Autodesk Inventor part; units mm, degrees
(part 2 of 2)
sketch "Sketch26" plane through (0, 0, 0) normal (0, -1, 0) x (1, 0, 0)
  circle A0 centre (0, 0) radius 28.575 construction
  spline S0 degree 2 poles (-30.0314, 4.4782) (-29.616, 4.4453) (-29.0046, 4.0789) (-28.8177, 3.8006) knots 0 0 0 1 2 2 2
  spline S1 degree 2 poles (-28.8177, 3.8006) (-28.5989, 3.4653) (-28.4482, 2.7311) (-28.4932, 2.1623) knots 0 0 0 1 2 2 2
  line L0 (-28.4932, 2.1623) -> (-28.6199, 0.5643)
  line L1 (-28.6199, 0.5643) -> (-34.1904, 1.0057)
  line L2 (-34.1904, 1.0057) -> (-34.0734, 2.4818)
  spline S2 degree 2 poles (-34.0734, 2.4818) (-34.0262, 3.0777) (-33.9023, 3.6675) (-33.7318, 3.9265) knots 0 0 0 1 2 2 2
  spline S3 degree 2 poles (-33.7318, 3.9265) (-33.5499, 4.2165) (-33.0089, 4.4507) (-32.6568, 4.4228) knots 0 0 0 1 2 2 2
  spline S4 degree 2 poles (-32.6568, 4.4228) (-32.2641, 4.3917) (-31.674, 3.927) (-31.5269, 3.5474) knots 0 0 0 1 2 2 2
  line L3 (-31.5269, 3.5474) -> (-31.4998, 3.5453)
  spline S5 degree 2 poles (-31.4998, 3.5453) (-31.3251, 4.0311) (-30.564, 4.5204) (-30.0314, 4.4782) knots 0 0 0 1 2 2 2
  spline S6 degree 2 poles (-30.0609, 3.7038) (-30.3769, 3.7288) (-30.7975, 3.5805) (-30.9634, 3.3211) knots 0 0 0 1 2 2 2
  spline S7 degree 2 poles (-30.9634, 3.3211) (-31.0676, 3.1522) (-31.1547, 2.7411) (-31.1851, 2.3574) knots 0 0 0 1 2 2 2
  line L4 (-31.1851, 2.3574) -> (-31.2517, 1.5178)
  line L5 (-31.2517, 1.5178) -> (-29.1932, 1.3547)
  line L6 (-29.1932, 1.3547) -> (-29.1456, 1.9551)
  spline S8 degree 2 poles (-29.1456, 1.9551) (-29.107, 2.4426) (-29.1529, 3.0095) (-29.2802, 3.2377) knots 0 0 0 1 2 2 2
  spline S9 degree 2 poles (-29.2802, 3.2377) (-29.4127, 3.4571) (-29.7675, 3.6806) (-30.0609, 3.7038) knots 0 0 0 1 2 2 2
  spline S10 degree 2 poles (-32.6141, 3.6426) (-32.8128, 3.6584) (-33.1214, 3.5466) (-33.219, 3.4044) knots 0 0 0 1 2 2 2
  spline S11 degree 2 poles (-33.219, 3.4044) (-33.3326, 3.2317) (-33.4125, 2.7974) (-33.4436, 2.4047) knots 0 0 0 1 2 2 2
  line L7 (-33.4436, 2.4047) -> (-33.4997, 1.6959)
  line L8 (-33.4997, 1.6959) -> (-31.8701, 1.5668)
  line L9 (-31.8701, 1.5668) -> (-31.8036, 2.4064)
  spline S12 degree 2 poles (-31.8036, 2.4064) (-31.776, 2.754) (-31.8222, 3.0893) (-31.9211, 3.2743) knots 0 0 0 1 2 2 2
  spline S13 degree 2 poles (-31.9211, 3.2743) (-32.0158, 3.4544) (-32.3523, 3.6219) (-32.6141, 3.6426) knots 0 0 0 1 2 2 2
  spline S14 degree 2 poles (-29.4283, 8.8448) (-28.3968, 8.6022) (-27.506, 7.346) (-27.7009, 6.5173) knots 0 0 0 1 2 2 2
  spline S15 degree 2 poles (-27.7009, 6.5173) (-27.901, 5.6665) (-29.2895, 4.965) (-30.2857, 5.1993) knots 0 0 0 1 2 2 2
  spline S16 degree 2 poles (-30.2857, 5.1993) (-31.3084, 5.4398) (-32.2049, 6.7113) (-32.012, 7.5312) knots 0 0 0 1 2 2 2
  spline S17 degree 2 poles (-32.012, 7.5312) (-31.8171, 8.3599) (-30.4554, 9.0863) (-29.4283, 8.8448) knots 0 0 0 1 2 2 2
  spline S18 degree 2 poles (-29.5952, 8.1351) (-30.3887, 8.3217) (-31.2959, 7.9256) (-31.4214, 7.3923) knots 0 0 0 1 2 2 2
  spline S19 degree 2 poles (-31.4214, 7.3923) (-31.5468, 6.8589) (-30.9122, 6.0956) (-30.1188, 5.909) knots 0 0 0 1 2 2 2
  spline S20 degree 2 poles (-30.1188, 5.909) (-29.3474, 5.7275) (-28.4171, 6.1228) (-28.2916, 6.6562) knots 0 0 0 1 2 2 2
  spline S21 degree 2 poles (-28.2916, 6.6562) (-28.1672, 7.1851) (-28.8106, 7.9505) (-29.5952, 8.1351) knots 0 0 0 1 2 2 2
  spline S22 degree 2 poles (-26.6089, 10.2025) (-26.8054, 9.662) (-27.6438, 9.2779) (-28.312, 9.5208) knots 0 0 0 1 2 2 2
  line L10 (-28.312, 9.5208) -> (-30.4951, 10.3148)
  line L11 (-30.4951, 10.3148) -> (-30.6576, 9.868)
  line L12 (-30.6576, 9.868) -> (-31.2066, 10.0676)
  line L13 (-31.2066, 10.0676) -> (-31.0441, 10.5145)
  line L14 (-31.0441, 10.5145) -> (-32.1761, 10.9262)
  line L15 (-32.1761, 10.9262) -> (-31.9347, 11.5901)
  line L16 (-31.9347, 11.5901) -> (-30.8027, 11.1784)
  line L17 (-30.8027, 11.1784) -> (-30.3585, 12.3997)
  line L18 (-30.3585, 12.3997) -> (-29.8095, 12.2001)
  line L19 (-29.8095, 12.2001) -> (-30.2537, 10.9787)
  line L20 (-30.2537, 10.9787) -> (-28.3769, 10.2962)
  spline S23 degree 2 poles (-28.3769, 10.2962) (-28.079, 10.1878) (-27.7436, 10.0899) (-27.5769, 10.1112) knots 0 0 0 1 2 2 2
  spline S24 degree 2 poles (-27.5769, 10.1112) (-27.4318, 10.1259) (-27.2109, 10.3491) (-27.1273, 10.5789) knots 0 0 0 1 2 2 2
  spline S25 degree 2 poles (-27.1273, 10.5789) (-27.0685, 10.7406) (-27.0565, 11.0784) (-27.0615, 11.1573) knots 0 0 0 1 2 2 2
  line L21 (-27.0615, 11.1573) -> (-27.0476, 11.1956)
  line L22 (-27.0476, 11.1956) -> (-26.4518, 10.9789)
  spline S26 degree 2 poles (-26.4518, 10.9789) (-26.4688, 10.7731) (-26.5485, 10.3684) (-26.6089, 10.2025) knots 0 0 0 1 2 2 2
  spline S27 degree 2 poles (-25.5848, 12.5515) (-25.8291, 12.0309) (-26.6986, 11.7236) (-27.3422, 12.0256) knots 0 0 0 1 2 2 2
  line L23 (-27.3422, 12.0256) -> (-29.4452, 13.0125)
  line L24 (-29.4452, 13.0125) -> (-29.6472, 12.5821)
  line L25 (-29.6472, 12.5821) -> (-30.1761, 12.8302)
  line L26 (-30.1761, 12.8302) -> (-29.9741, 13.2607)
  line L27 (-29.9741, 13.2607) -> (-31.0645, 13.7724)
  line L28 (-31.0645, 13.7724) -> (-30.7644, 14.4119)
  line L29 (-30.7644, 14.4119) -> (-29.674, 13.9002)
  line L30 (-29.674, 13.9002) -> (-29.1219, 15.0767)
  line L31 (-29.1219, 15.0767) -> (-28.593, 14.8286)
  line L32 (-28.593, 14.8286) -> (-29.1451, 13.652)
  line L33 (-29.1451, 13.652) -> (-27.3373, 12.8037)
  spline S28 degree 2 poles (-27.3373, 12.8037) (-27.0503, 12.669) (-26.7251, 12.5414) (-26.5571, 12.5476) knots 0 0 0 1 2 2 2
  spline S29 degree 2 poles (-26.5571, 12.5476) (-26.4113, 12.5492) (-26.1712, 12.7516) (-26.0673, 12.973) knots 0 0 0 1 2 2 2
  spline S30 degree 2 poles (-26.0673, 12.973) (-25.9942, 13.1288) (-25.9519, 13.4641) (-25.9498, 13.5432) knots 0 0 0 1 2 2 2
  line L34 (-25.9498, 13.5432) -> (-25.9325, 13.58)
  line L35 (-25.9325, 13.58) -> (-25.3586, 13.3107)
  spline S31 degree 2 poles (-25.3586, 13.3107) (-25.394, 13.1073) (-25.5098, 12.7114) (-25.5848, 12.5515) knots 0 0 0 1 2 2 2
  spline S32 degree 2 poles (-25.0529, 17.7935) (-24.1532, 17.2337) (-23.711, 15.7585) (-24.1608, 15.0357) knots 0 0 0 1 2 2 2
  spline S33 degree 2 poles (-24.1608, 15.0357) (-24.6225, 14.2936) (-26.1624, 14.0731) (-27.0313, 14.6138) knots 0 0 0 1 2 2 2
  spline S34 degree 2 poles (-27.0313, 14.6138) (-27.9233, 15.1688) (-28.366, 16.6602) (-27.9211, 17.3754) knots 0 0 0 1 2 2 2
  spline S35 degree 2 poles (-27.9211, 17.3754) (-27.4713, 18.0982) (-25.9488, 18.3509) (-25.0529, 17.7935) knots 0 0 0 1 2 2 2
  spline S36 degree 2 poles (-25.4381, 17.1744) (-26.1301, 17.6051) (-27.1164, 17.52) (-27.4058, 17.0548) knots 0 0 0 1 2 2 2
  spline S37 degree 2 poles (-27.4058, 17.0548) (-27.6953, 16.5896) (-27.3382, 15.6634) (-26.6462, 15.2328) knots 0 0 0 1 2 2 2
  spline S38 degree 2 poles (-26.6462, 15.2328) (-25.9733, 14.8141) (-24.9655, 14.891) (-24.676, 15.3563) knots 0 0 0 1 2 2 2
  spline S39 degree 2 poles (-24.676, 15.3563) (-24.3889, 15.8177) (-24.7537, 16.7486) (-25.4381, 17.1744) knots 0 0 0 1 2 2 2
  line L36 (-19.6872, 20.8112) -> (-21.4766, 22.4512)
  spline S40 degree 2 poles (-21.4766, 22.4512) (-21.6902, 22.647) (-22.0847, 22.9471) (-22.2338, 22.9855) knots 0 0 0 1 2 2 2
  spline S41 degree 2 poles (-22.2338, 22.9855) (-22.3929, 23.033) (-22.6864, 22.9273) (-22.8486, 22.7504) knots 0 0 0 1 2 2 2
  spline S42 degree 2 poles (-22.8486, 22.7504) (-22.9954, 22.5901) (-23.135, 22.0424) (-23.1255, 21.6774) knots 0 0 0 1 2 2 2
  spline S43 degree 2 poles (-23.1255, 21.6774) (-23.0758, 21.6379) (-22.9394, 21.5253) (-22.8526, 21.4457) knots 0 0 0 1 2 2 2
  line L37 (-22.8526, 21.4457) -> (-20.8163, 19.5793)
  line L38 (-20.8163, 19.5793) -> (-21.2936, 19.0586)
  line L39 (-21.2936, 19.0586) -> (-23.0829, 20.6985)
  spline S44 degree 2 poles (-23.0829, 20.6985) (-23.2966, 20.8944) (-23.691, 21.1945) (-23.8401, 21.2329) knots 0 0 0 1 2 2 2
  spline S45 degree 2 poles (-23.8401, 21.2329) (-23.9993, 21.2804) (-24.2927, 21.1747) (-24.4549, 20.9978) knots 0 0 0 1 2 2 2
  spline S46 degree 2 poles (-24.4549, 20.9978) (-24.6079, 20.8308) (-24.7372, 20.2675) (-24.7327, 19.944) knots 0 0 0 1 2 2 2
  line L40 (-24.7327, 19.944) -> (-22.4226, 17.8267)
  line L41 (-22.4226, 17.8267) -> (-22.8999, 17.3059)
  line L42 (-22.8999, 17.3059) -> (-25.9912, 20.1392)
  line L43 (-25.9912, 20.1392) -> (-25.5139, 20.66)
  line L44 (-25.5139, 20.66) -> (-25.1734, 20.3479)
  spline S47 degree 2 poles (-25.1734, 20.3479) (-25.1904, 20.7382) (-25.0469, 21.3438) (-24.8266, 21.5841) knots 0 0 0 1 2 2 2
  spline S48 degree 2 poles (-24.8266, 21.5841) (-24.5757, 21.8579) (-23.9367, 22.0524) (-23.552, 21.9024) knots 0 0 0 1 2 2 2
  spline S49 degree 2 poles (-23.552, 21.9024) (-23.5985, 22.3812) (-23.4589, 23.0764) (-23.2203, 23.3367) knots 0 0 0 1 2 2 2
  spline S50 degree 2 poles (-23.2203, 23.3367) (-23.0367, 23.537) (-22.6133, 23.751) (-22.3629, 23.7427) knots 0 0 0 1 2 2 2
  spline S51 degree 2 poles (-22.3629, 23.7427) (-22.1095, 23.7377) (-21.5635, 23.489) (-21.2463, 23.1984) knots 0 0 0 1 2 2 2
  line L45 (-21.2463, 23.1984) -> (-19.2099, 21.332)
  line L46 (-19.2099, 21.332) -> (-19.6872, 20.8112)
  line L47 (-13.0022, 25.5262) -> (-13.6384, 25.1431)
  line L48 (-13.6384, 25.1431) -> (-15.0493, 27.4863)
  line L49 (-15.0493, 27.4863) -> (-17.2528, 26.1595)
  line L50 (-17.2528, 26.1595) -> (-15.8419, 23.8163)
  line L51 (-15.8419, 23.8163) -> (-16.4781, 23.4332)
  line L52 (-16.4781, 23.4332) -> (-19.3607, 28.2204)
  line L53 (-19.3607, 28.2204) -> (-18.7245, 28.6035)
  line L54 (-18.7245, 28.6035) -> (-17.5939, 26.7259)
  line L55 (-17.5939, 26.7259) -> (-15.3904, 28.0527)
  line L56 (-15.3904, 28.0527) -> (-16.521, 29.9303)
  line L57 (-16.521, 29.9303) -> (-15.8847, 30.3134)
  line L58 (-15.8847, 30.3134) -> (-13.0022, 25.5262)
  spline S52 degree 2 poles (-10.2968, 26.5552) (-11.2301, 26.1816) (-12.6749, 26.8177) (-13.062, 27.7846) knots 0 0 0 1 2 2 2
  spline S53 degree 2 poles (-13.062, 27.7846) (-13.4424, 28.7347) (-12.8971, 30.2603) (-12.0941, 30.5817) knots 0 0 0 1 2 2 2
  spline S54 degree 2 poles (-12.0941, 30.5817) (-11.7325, 30.7265) (-11.0893, 30.7401) (-10.7941, 30.5997) knots 0 0 0 1 2 2 2
  spline S55 degree 2 poles (-10.7941, 30.5997) (-10.4947, 30.4611) (-10.0144, 29.9071) (-9.8275, 29.4404) knots 0 0 0 1 2 2 2
  line L59 (-9.8275, 29.4404) -> (-9.6845, 29.0831)
  line L60 (-9.6845, 29.0831) -> (-12.3793, 28.0043)
  spline S56 degree 2 poles (-12.3793, 28.0043) (-12.1083, 27.3274) (-11.1395, 26.8812) (-10.5341, 27.1236) knots 0 0 0 1 2 2 2
  spline S57 degree 2 poles (-10.5341, 27.1236) (-10.3197, 27.2094) (-9.9422, 27.4727) (-9.8043, 27.6157) knots 0 0 0 1 2 2 2
  spline S58 degree 2 poles (-9.8043, 27.6157) (-9.6614, 27.7705) (-9.4765, 28.0152) (-9.4235, 28.1145) knots 0 0 0 1 2 2 2
  line L61 (-9.4235, 28.1145) -> (-9.3857, 28.1296)
  line L62 (-9.3857, 28.1296) -> (-9.0996, 27.4149)
  spline S59 degree 2 poles (-9.0996, 27.4149) (-9.1946, 27.3232) (-9.4855, 27.0507) (-9.6048, 26.959) knots 0 0 0 1 2 2 2
  spline S60 degree 2 poles (-9.6048, 26.959) (-9.7721, 26.8286) (-10.0614, 26.6494) (-10.2968, 26.5552) knots 0 0 0 1 2 2 2
  spline S61 degree 2 poles (-10.5238, 29.3275) (-10.6382, 29.589) (-10.9024, 29.932) (-11.0596, 30.0203) knots 0 0 0 1 2 2 2
  spline S62 degree 2 poles (-11.0596, 30.0203) (-11.232, 30.122) (-11.6516, 30.1345) (-11.9165, 30.0285) knots 0 0 0 1 2 2 2
  spline S63 degree 2 poles (-11.9165, 30.0285) (-12.1771, 29.9241) (-12.4806, 29.6221) (-12.5714, 29.4102) knots 0 0 0 1 2 2 2
  spline S64 degree 2 poles (-12.5714, 29.4102) (-12.6562, 29.1958) (-12.6578, 28.761) (-12.5795, 28.5046) knots 0 0 0 1 2 2 2
  line L63 (-12.5795, 28.5046) -> (-10.5238, 29.3275)
  line L64 (-5.0842, 28.1809) -> (-5.9236, 27.9722)
  line L65 (-5.9236, 27.9722) -> (-7.2926, 29.2557)
  line L66 (-7.2926, 29.2557) -> (-7.9275, 27.4739)
  line L67 (-7.9275, 27.4739) -> (-8.7053, 27.2805)
  line L68 (-8.7053, 27.2805) -> (-7.7962, 29.6484)
  line L69 (-7.7962, 29.6484) -> (-9.7039, 31.3532)
  line L70 (-9.7039, 31.3532) -> (-8.8646, 31.5619)
  line L71 (-8.8646, 31.5619) -> (-7.5032, 30.2905)
  line L72 (-7.5032, 30.2905) -> (-6.8738, 32.0569)
  line L73 (-6.8738, 32.0569) -> (-6.096, 32.2503)
  line L74 (-6.096, 32.2503) -> (-6.9985, 29.8934)
  line L75 (-6.9985, 29.8934) -> (-5.0842, 28.1809)
  line L76 (-3.6562, 31.4912) -> (-4.5453, 31.3752)
  line L77 (-4.5453, 31.3752) -> (-4.6835, 32.4349)
  line L78 (-4.6835, 32.4349) -> (-3.7944, 32.5509)
  line L79 (-3.7944, 32.5509) -> (-3.6562, 31.4912)
  line L80 (-3.252, 28.3929) -> (-4.1411, 28.2769)
  line L81 (-4.1411, 28.2769) -> (-4.2793, 29.3366)
  line L82 (-4.2793, 29.3366) -> (-3.3902, 29.4526)
  line L83 (-3.3902, 29.4526) -> (-3.252, 28.3929)
  spline S65 degree 2 poles (4.133, 31.1469) (4.0204, 29.6477) (3.0434, 28.3088) (2.1358, 28.377) knots 0 0 0 1 2 2 2
  spline S66 degree 2 poles (2.1358, 28.377) (1.2146, 28.4462) (0.4596, 29.9424) (0.5698, 31.41) knots 0 0 0 1 2 2 2
  spline S67 degree 2 poles (0.5698, 31.41) (0.6831, 32.9182) (1.6594, 34.2481) (2.5716, 34.1796) knots 0 0 0 1 2 2 2
  spline S68 degree 2 poles (2.5716, 34.1796) (3.4883, 34.1108) (4.2422, 32.601) (4.133, 31.1469) knots 0 0 0 1 2 2 2
  spline S69 degree 2 poles (3.0482, 29.521) (3.1772, 29.7883) (3.3313, 30.6304) (3.3744, 31.2039) knots 0 0 0 1 2 2 2
  spline S70 degree 2 poles (3.3744, 31.2039) (3.4175, 31.7774) (3.3906, 32.6286) (3.299, 32.9216) knots 0 0 0 1 2 2 2
  spline S71 degree 2 poles (3.299, 32.9216) (3.2075, 33.2145) (2.8367, 33.5376) (2.5251, 33.561) knots 0 0 0 1 2 2 2
  spline S72 degree 2 poles (2.5251, 33.561) (2.2135, 33.5844) (1.7896, 33.321) (1.6501, 33.0363) knots 0 0 0 1 2 2 2
  spline S73 degree 2 poles (1.6501, 33.0363) (1.5159, 32.7603) (1.3695, 31.8994) (1.3285, 31.353) knots 0 0 0 1 2 2 2
  spline S74 degree 2 poles (1.3285, 31.353) (1.2844, 30.766) (1.2976, 29.9748) (1.392, 29.659) knots 0 0 0 1 2 2 2
  spline S75 degree 2 poles (1.392, 29.659) (1.4786, 29.3618) (1.8571, 29.0201) (2.1822, 28.9956) knots 0 0 0 1 2 2 2
  spline S76 degree 2 poles (2.1822, 28.9956) (2.4893, 28.9726) (2.9132, 29.2359) (3.0482, 29.521) knots 0 0 0 1 2 2 2
  line L84 (5.8019, 27.9833) -> (4.9213, 28.1517)
  line L85 (4.9213, 28.1517) -> (5.122, 29.2014)
  line L86 (5.122, 29.2014) -> (6.0026, 29.033)
  line L87 (6.0026, 29.033) -> (5.8019, 27.9833)
  spline S77 degree 2 poles (10.6727, 28.4624) (10.5525, 28.0777) (10.1009, 27.4977) (9.8005, 27.3259) knots 0 0 0 1 2 2 2
  spline S78 degree 2 poles (9.8005, 27.3259) (9.5001, 27.154) (8.7424, 27.0824) (8.3274, 27.2121) knots 0 0 0 1 2 2 2
  spline S79 degree 2 poles (8.3274, 27.2121) (7.9471, 27.3309) (7.2563, 27.7318) (7.0259, 27.9509) knots 0 0 0 1 2 2 2
  line L88 (7.0259, 27.9509) -> (7.2622, 28.7073)
  line L89 (7.2622, 28.7073) -> (7.3141, 28.6911)
  spline S80 degree 2 poles (7.3141, 28.6911) (7.3773, 28.6049) (7.6356, 28.3534) (7.7998, 28.2262) knots 0 0 0 1 2 2 2
  spline S81 degree 2 poles (7.7998, 28.2262) (7.9886, 28.0865) (8.3131, 27.895) (8.5335, 27.8261) knots 0 0 0 1 2 2 2
  spline S82 degree 2 poles (8.5335, 27.8261) (8.7496, 27.7586) (9.2045, 27.7872) (9.4042, 27.9099) knots 0 0 0 1 2 2 2
  spline S83 degree 2 poles (9.4042, 27.9099) (9.5881, 28.028) (9.8588, 28.4083) (9.9479, 28.6936) knots 0 0 0 1 2 2 2
  spline S84 degree 2 poles (9.9479, 28.6936) (10.0371, 28.9789) (9.9949, 29.3905) (9.8858, 29.5575) knots 0 0 0 1 2 2 2
  spline S85 degree 2 poles (9.8858, 29.5575) (9.7764, 29.7387) (9.362, 29.9916) (9.0897, 30.0767) knots 0 0 0 1 2 2 2
  spline S86 degree 2 poles (9.0897, 30.0767) (8.7958, 30.1685) (8.1839, 30.2601) (7.9945, 30.2765) knots 0 0 0 1 2 2 2
  line L90 (7.9945, 30.2765) -> (8.8535, 33.0255)
  line L91 (8.8535, 33.0255) -> (11.7797, 32.1112)
  line L92 (11.7797, 32.1112) -> (11.5838, 31.4844)
  line L93 (11.5838, 31.4844) -> (9.3449, 32.184)
  line L94 (9.3449, 32.184) -> (8.9006, 30.762)
  spline S87 degree 2 poles (8.9006, 30.762) (9.0356, 30.7388) (9.2904, 30.6734) (9.3941, 30.641) knots 0 0 0 1 2 2 2
  spline S88 degree 2 poles (9.3941, 30.641) (9.8047, 30.5127) (10.3291, 30.2018) (10.5263, 29.9219) knots 0 0 0 1 2 2 2
  spline S89 degree 2 poles (10.5263, 29.9219) (10.7278, 29.6407) (10.824, 28.9465) (10.6727, 28.4624) knots 0 0 0 1 2 2 2
  line L95 (13.9948, 24.9753) -> (10.8908, 26.4722)
  line L96 (10.8908, 26.4722) -> (11.235, 27.186)
  spline S90 degree 2 poles (11.235, 27.186) (11.7209, 27.3387) (12.5977, 27.6348) (13.0347, 27.8112) knots 0 0 0 1 2 2 2
  spline S91 degree 2 poles (13.0347, 27.8112) (13.9147, 28.1661) (14.7007, 28.7221) (14.8954, 29.126) knots 0 0 0 1 2 2 2
  spline S92 degree 2 poles (14.8954, 29.126) (14.9977, 29.3381) (15.0206, 29.7191) (14.9515, 29.8782) knots 0 0 0 1 2 2 2
  spline S93 degree 2 poles (14.9515, 29.8782) (14.8824, 30.0372) (14.6215, 30.2886) (14.4339, 30.3791) knots 0 0 0 1 2 2 2
  spline S94 degree 2 poles (14.4339, 30.3791) (14.2544, 30.4657) (13.8441, 30.553) (13.6434, 30.5643) knots 0 0 0 1 2 2 2
  spline S95 degree 2 poles (13.6434, 30.5643) (13.4731, 30.576) (13.1293, 30.5407) (13.0202, 30.5229) knots 0 0 0 1 2 2 2
  line L97 (13.0202, 30.5229) -> (12.9835, 30.5407)
  line L98 (12.9835, 30.5407) -> (13.3297, 31.2585)
  spline S96 degree 2 poles (13.3297, 31.2585) (13.5869, 31.2602) (14.4297, 31.1001) (14.7641, 30.9388) knots 0 0 0 1 2 2 2
  spline S97 degree 2 poles (14.7641, 30.9388) (15.4698, 30.5985) (15.9052, 29.4685) (15.5983, 28.8322) knots 0 0 0 1 2 2 2
  spline S98 degree 2 poles (15.5983, 28.8322) (15.4548, 28.5345) (15.0761, 28.1037) (14.8514, 27.9506) knots 0 0 0 1 2 2 2
  spline S99 degree 2 poles (14.8514, 27.9506) (14.6229, 27.7894) (14.0595, 27.5281) (13.7634, 27.4145) knots 0 0 0 1 2 2 2
  spline S100 degree 2 poles (13.7634, 27.4145) (13.2781, 27.2213) (12.141, 26.8546) (11.8043, 26.7505) knots 0 0 0 1 2 2 2
  line L99 (11.8043, 26.7505) -> (14.276, 25.5585)
  line L100 (14.276, 25.5585) -> (13.9948, 24.9753)
  line L101 (17.4903, 22.6651) -> (14.638, 24.599)
  line L102 (14.638, 24.599) -> (15.0827, 25.2549)
  spline S101 degree 2 poles (15.0827, 25.2549) (15.5857, 25.3352) (16.4964, 25.5001) (16.9544, 25.6108) knots 0 0 0 1 2 2 2
  spline S102 degree 2 poles (16.9544, 25.6108) (17.8768, 25.8335) (18.7355, 26.2688) (18.9871, 26.6399) knots 0 0 0 1 2 2 2
  spline S103 degree 2 poles (18.9871, 26.6399) (19.1192, 26.8348) (19.1975, 27.2085) (19.1524, 27.3759) knots 0 0 0 1 2 2 2
  spline S104 degree 2 poles (19.1524, 27.3759) (19.1072, 27.5433) (18.8859, 27.8301) (18.7135, 27.947) knots 0 0 0 1 2 2 2
  spline S105 degree 2 poles (18.7135, 27.947) (18.5486, 28.0588) (18.1553, 28.2051) (17.9584, 28.2456) knots 0 0 0 1 2 2 2
  spline S106 degree 2 poles (17.9584, 28.2456) (17.7917, 28.282) (17.4464, 28.2973) (17.3359, 28.2956) knots 0 0 0 1 2 2 2
  line L103 (17.3359, 28.2956) -> (17.3021, 28.3185)
  line L104 (17.3021, 28.3185) -> (17.7494, 28.9782)
  spline S107 degree 2 poles (17.7494, 28.9782) (18.0041, 28.9423) (18.8145, 28.6609) (19.1218, 28.4525) knots 0 0 0 1 2 2 2
  spline S108 degree 2 poles (19.1218, 28.4525) (19.7703, 28.0128) (20.0361, 26.8314) (19.6396, 26.2467) knots 0 0 0 1 2 2 2
  spline S109 degree 2 poles (19.6396, 26.2467) (19.4541, 25.9731) (19.0167, 25.6022) (18.7721, 25.4836) knots 0 0 0 1 2 2 2
  spline S110 degree 2 poles (18.7721, 25.4836) (18.5224, 25.3574) (17.9269, 25.1812) (17.6174, 25.112) knots 0 0 0 1 2 2 2
  spline S111 degree 2 poles (17.6174, 25.112) (17.1091, 24.9917) (15.9307, 24.7949) (15.5824, 24.7411) knots 0 0 0 1 2 2 2
  line L105 (15.5824, 24.7411) -> (17.8537, 23.2011)
  line L106 (17.8537, 23.2011) -> (17.4903, 22.6651)
  spline S112 degree 2 poles (21.7678, 21.2174) (21.4953, 20.9204) (20.8398, 20.5877) (20.4949, 20.56) knots 0 0 0 1 2 2 2
  spline S113 degree 2 poles (20.4949, 20.56) (20.1499, 20.5323) (19.4337, 20.7899) (19.1134, 21.0837) knots 0 0 0 1 2 2 2
  spline S114 degree 2 poles (19.1134, 21.0837) (18.8197, 21.3531) (18.3651, 22.0098) (18.2498, 22.3061) knots 0 0 0 1 2 2 2
  line L107 (18.2498, 22.3061) -> (18.7855, 22.89)
  line L108 (18.7855, 22.89) -> (18.8255, 22.8533)
  spline S115 degree 2 poles (18.8255, 22.8533) (18.8461, 22.7484) (18.9728, 22.4109) (19.0673, 22.2259) knots 0 0 0 1 2 2 2
  spline S116 degree 2 poles (19.0673, 22.2259) (19.1788, 22.0192) (19.3909, 21.7079) (19.5611, 21.5517) knots 0 0 0 1 2 2 2
  spline S117 degree 2 poles (19.5611, 21.5517) (19.728, 21.3987) (20.1518, 21.2311) (20.3847, 21.2571) knots 0 0 0 1 2 2 2
  spline S118 degree 2 poles (20.3847, 21.2571) (20.6014, 21.2857) (21.0082, 21.5148) (21.2102, 21.735) knots 0 0 0 1 2 2 2
  spline S119 degree 2 poles (21.2102, 21.735) (21.4122, 21.9553) (21.5492, 22.3458) (21.5215, 22.5433) knots 0 0 0 1 2 2 2
  spline S120 degree 2 poles (21.5215, 22.5433) (21.4996, 22.7539) (21.2321, 23.159) (21.0219, 23.3518) knots 0 0 0 1 2 2 2
  spline S121 degree 2 poles (21.0219, 23.3518) (20.795, 23.56) (20.2802, 23.9032) (20.1158, 23.9986) knots 0 0 0 1 2 2 2
  line L109 (20.1158, 23.9986) -> (22.0627, 26.121)
  line L110 (22.0627, 26.121) -> (24.3219, 24.0486)
  line L111 (24.3219, 24.0486) -> (23.878, 23.5647)
  line L112 (23.878, 23.5647) -> (22.1494, 25.1504)
  line L113 (22.1494, 25.1504) -> (21.1423, 24.0525)
  spline S122 degree 2 poles (21.1423, 24.0525) (21.2547, 23.974) (21.4574, 23.8065) (21.5375, 23.733) knots 0 0 0 1 2 2 2
  spline S123 degree 2 poles (21.5375, 23.733) (21.8545, 23.4422) (22.1968, 22.9378) (22.2562, 22.6006) knots 0 0 0 1 2 2 2
  spline S124 degree 2 poles (22.2562, 22.6006) (22.3189, 22.2604) (22.1106, 21.5912) (21.7678, 21.2174) knots 0 0 0 1 2 2 2
  line L114 (23.8654, 15.7525) -> (22.6056, 17.5127)
  line L115 (22.6056, 17.5127) -> (23.0696, 17.8448)
  line L116 (23.0696, 17.8448) -> (23.4833, 17.2666)
  line L117 (23.4833, 17.2666) -> (27.0994, 19.8547)
  line L118 (27.0994, 19.8547) -> (26.6857, 20.4329)
  line L119 (26.6857, 20.4329) -> (27.1497, 20.7649)
  line L120 (27.1497, 20.7649) -> (28.4094, 19.0048)
  line L121 (28.4094, 19.0048) -> (27.9455, 18.6727)
  line L122 (27.9455, 18.6727) -> (27.5317, 19.2508)
  line L123 (27.5317, 19.2508) -> (23.9156, 16.6627)
  line L124 (23.9156, 16.6627) -> (24.3293, 16.0846)
  line L125 (24.3293, 16.0846) -> (23.8654, 15.7525)
  spline S125 degree 2 poles (28.9112, 12.3884) (28.2324, 12.035) (26.8534, 12.0163) (26.3076, 12.3192) knots 0 0 0 1 2 2 2
  spline S126 degree 2 poles (26.3076, 12.3192) (25.874, 12.5733) (25.3097, 13.2648) (24.9959, 13.8673) knots 0 0 0 1 2 2 2
  line L126 (24.9959, 13.8673) -> (24.4019, 15.0079)
  line L127 (24.4019, 15.0079) -> (29.3581, 17.589)
  line L128 (29.3581, 17.589) -> (29.9459, 16.4604)
  spline S127 degree 2 poles (29.9459, 16.4604) (30.3098, 15.7615) (30.5151, 14.8575) (30.4768, 14.4802) knots 0 0 0 1 2 2 2
  spline S128 degree 2 poles (30.4768, 14.4802) (30.4084, 13.837) (29.6341, 12.7649) (28.9112, 12.3884) knots 0 0 0 1 2 2 2
  spline S129 degree 2 poles (28.5615, 13.0794) (29.1318, 13.3764) (29.7425, 14.1744) (29.7769, 14.6671) knots 0 0 0 1 2 2 2
  spline S130 degree 2 poles (29.7769, 14.6671) (29.7955, 15.0138) (29.6245, 15.6854) (29.3923, 16.1312) knots 0 0 0 1 2 2 2
  line L129 (29.3923, 16.1312) -> (29.1308, 16.6333)
  line L130 (29.1308, 16.6333) -> (25.3153, 14.6463)
  line L131 (25.3153, 14.6463) -> (25.5767, 14.1442)
  spline S131 degree 2 poles (25.5767, 14.1442) (25.8047, 13.7064) (26.2904, 13.1169) (26.6193, 12.9461) knots 0 0 0 1 2 2 2
  spline S132 degree 2 poles (26.6193, 12.9461) (27.0321, 12.7221) (27.9832, 12.7782) (28.5615, 13.0794) knots 0 0 0 1 2 2 2
  line L132 (30.0174, 10.1989) -> (29.717, 11.0437)
  line L133 (29.717, 11.0437) -> (30.7239, 11.4018)
  line L134 (30.7239, 11.4018) -> (31.0243, 10.557)
  line L135 (31.0243, 10.557) -> (30.0174, 10.1989)
  line L136 (27.0735, 9.152) -> (26.773, 9.9968)
  line L137 (26.773, 9.9968) -> (27.78, 10.3549)
  line L138 (27.78, 10.3549) -> (28.0804, 9.5101)
  line L139 (28.0804, 9.5101) -> (27.0735, 9.152)
  line L140 (28.5089, 2.4396) -> (28.1367, 5.1402)
  line L141 (28.1367, 5.1402) -> (28.7019, 5.2181)
  line L142 (28.7019, 5.2181) -> (28.8404, 4.2132)
  line L143 (28.8404, 4.2132) -> (32.5503, 4.7246)
  line L144 (32.5503, 4.7246) -> (32.4118, 5.7295)
  line L145 (32.4118, 5.7295) -> (32.9187, 5.7993)
  spline S133 degree 2 poles (32.9187, 5.7993) (32.9972, 5.2296) (33.3944, 4.7358) (33.8479, 4.7618) knots 0 0 0 1 2 2 2
  line L146 (33.8479, 4.7618) -> (33.9271, 4.1876)
  line L147 (33.9271, 4.1876) -> (28.9387, 3.5)
  line L148 (28.9387, 3.5) -> (29.0741, 2.5175)
  line L149 (29.0741, 2.5175) -> (28.5089, 2.4396)
  line L150 (28.5776, 0.2145) -> (28.557, 1.1109)
  line L151 (28.557, 1.1109) -> (29.6254, 1.1355)
  line L152 (29.6254, 1.1355) -> (29.6461, 0.2391)
  line L153 (29.6461, 0.2391) -> (28.5776, 0.2145)
  spline S134 degree 2 poles (30.0706, -4.4465) (29.6693, -4.4099) (29.0072, -4.0904) (28.7761, -3.8328) knots 0 0 0 1 2 2 2
  spline S135 degree 2 poles (28.7761, -3.8328) (28.5449, -3.5753) (28.3155, -2.8496) (28.355, -2.4167) knots 0 0 0 1 2 2 2
  spline S136 degree 2 poles (28.355, -2.4167) (28.3911, -2.0198) (28.6377, -1.2602) (28.8034, -0.9888) knots 0 0 0 1 2 2 2
  line L154 (28.8034, -0.9888) -> (29.5926, -1.0608)
  line L155 (29.5926, -1.0608) -> (29.5877, -1.1149)
  spline S137 degree 2 poles (29.5877, -1.1149) (29.5167, -1.1948) (29.3252, -1.5002) (29.2354, -1.6875) knots 0 0 0 1 2 2 2
  spline S138 degree 2 poles (29.2354, -1.6875) (29.1386, -1.9015) (29.0196, -2.259) (28.9986, -2.489) knots 0 0 0 1 2 2 2
  spline S139 degree 2 poles (28.9986, -2.489) (28.9781, -2.7145) (29.1018, -3.1532) (29.2637, -3.3225) knots 0 0 0 1 2 2 2
  spline S140 degree 2 poles (29.2637, -3.3225) (29.4178, -3.4775) (29.8466, -3.6621) (30.1442, -3.6893) knots 0 0 0 1 2 2 2
  spline S141 degree 2 poles (30.1442, -3.6893) (30.4418, -3.7164) (30.8354, -3.5886) (30.9757, -3.4468) knots 0 0 0 1 2 2 2
  spline S142 degree 2 poles (30.9757, -3.4468) (31.1299, -3.3017) (31.2899, -2.8434) (31.3158, -2.5593) knots 0 0 0 1 2 2 2
  spline S143 degree 2 poles (31.3158, -2.5593) (31.3437, -2.2526) (31.3045, -1.6352) (31.2808, -1.4466) knots 0 0 0 1 2 2 2
  line L156 (31.2808, -1.4466) -> (34.149, -1.708)
  line L157 (34.149, -1.708) -> (33.8706, -4.7611)
  line L158 (33.8706, -4.7611) -> (33.2167, -4.7015)
  line L159 (33.2167, -4.7015) -> (33.4297, -2.3655)
  line L160 (33.4297, -2.3655) -> (31.946, -2.2302)
  spline S144 degree 2 poles (31.946, -2.2302) (31.9517, -2.3671) (31.9414, -2.6299) (31.9315, -2.7382) knots 0 0 0 1 2 2 2
  spline S145 degree 2 poles (31.9315, -2.7382) (31.8925, -3.1666) (31.6988, -3.7446) (31.4667, -3.9963) knots 0 0 0 1 2 2 2
  spline S146 degree 2 poles (31.4667, -3.9963) (31.2342, -4.2525) (30.5757, -4.4925) (30.0706, -4.4465) knots 0 0 0 1 2 2 2
  line L161 (33.6613, -7.155) -> (31.5744, -6.5256)
  line L162 (31.5744, -6.5256) -> (31.6812, -6.0437)
  line L163 (31.6812, -6.0437) -> (33.8386, -6.3548)
  line L164 (33.8386, -6.3548) -> (33.6613, -7.155)
  line L165 (33.3557, -8.5344) -> (31.2688, -7.905)
  line L166 (31.2688, -7.905) -> (31.3756, -7.4231)
  line L167 (31.3756, -7.4231) -> (33.533, -7.7342)
  line L168 (33.533, -7.7342) -> (33.3557, -8.5344)
  spline S147 degree 2 poles (29.3913, -16.226) (28.919, -16.3495) (27.7869, -16.1939) (27.1592, -15.8901) knots 0 0 0 1 2 2 2
  spline S148 degree 2 poles (27.1592, -15.8901) (26.5478, -15.5942) (25.7072, -14.805) (25.5151, -14.3497) knots 0 0 0 1 2 2 2
  spline S149 degree 2 poles (25.5151, -14.3497) (25.3145, -13.8703) (25.3768, -12.8892) (25.6155, -12.396) knots 0 0 0 1 2 2 2
  spline S150 degree 2 poles (25.6155, -12.396) (25.8621, -11.8865) (26.6031, -11.239) (27.0855, -11.1052) knots 0 0 0 1 2 2 2
  spline S151 degree 2 poles (27.0855, -11.1052) (27.5598, -10.9776) (28.692, -11.1433) (29.3116, -11.4432) knots 0 0 0 1 2 2 2
  spline S152 degree 2 poles (29.3116, -11.4432) (29.9434, -11.749) (30.7534, -12.5284) (30.9598, -12.9855) knots 0 0 0 1 2 2 2
  spline S153 degree 2 poles (30.9598, -12.9855) (31.152, -13.4408) (31.1019, -14.4278) (30.8572, -14.9332) knots 0 0 0 1 2 2 2
  spline S154 degree 2 poles (30.8572, -14.9332) (30.6087, -15.4468) (29.8514, -16.0965) (29.3913, -16.226) knots 0 0 0 1 2 2 2
  spline S155 degree 2 poles (27.4965, -15.1931) (27.9938, -15.4338) (28.8687, -15.5907) (29.2161, -15.5173) knots 0 0 0 1 2 2 2
  spline S156 degree 2 poles (29.2161, -15.5173) (29.5737, -15.4439) (30.1068, -15.0076) (30.2765, -14.6571) knots 0 0 0 1 2 2 2
  spline S157 degree 2 poles (30.2765, -14.6571) (30.4521, -14.2943) (30.4637, -13.6258) (30.2953, -13.2878) knots 0 0 0 1 2 2 2
  spline S158 degree 2 poles (30.2953, -13.2878) (30.1352, -12.9637) (29.4633, -12.3769) (28.9742, -12.1402) knots 0 0 0 1 2 2 2
  spline S159 degree 2 poles (28.9742, -12.1402) (27.9838, -11.6608) (26.5297, -11.9833) (26.1923, -12.6803) knots 0 0 0 1 2 2 2
  spline S160 degree 2 poles (26.1923, -12.6803) (25.855, -13.3773) (26.5061, -14.7137) (27.4965, -15.1931) knots 0 0 0 1 2 2 2
  spline S161 degree 2 poles (23.814, -20.548) (23.1986, -20.0931) (22.577, -18.862) (22.6098, -18.2386) knots 0 0 0 1 2 2 2
  spline S162 degree 2 poles (22.6098, -18.2386) (22.6481, -17.7375) (23.022, -16.9271) (23.4258, -16.3809) knots 0 0 0 1 2 2 2
  line L169 (23.4258, -16.3809) -> (24.1903, -15.3467)
  line L170 (24.1903, -15.3467) -> (28.6837, -18.6687)
  line L171 (28.6837, -18.6687) -> (27.9272, -19.6919)
  spline S163 degree 2 poles (27.9272, -19.6919) (27.4588, -20.3255) (26.7364, -20.9065) (26.3805, -21.0375) knots 0 0 0 1 2 2 2
  spline S164 degree 2 poles (26.3805, -21.0375) (25.7725, -21.2582) (24.4695, -21.0326) (23.814, -20.548) knots 0 0 0 1 2 2 2
  spline S165 degree 2 poles (24.2816, -19.9307) (24.7987, -20.313) (25.7837, -20.5118) (26.2416, -20.3266) knots 0 0 0 1 2 2 2
  spline S166 degree 2 poles (26.2416, -20.3266) (26.5613, -20.1913) (27.0898, -19.7429) (27.3886, -19.3387) knots 0 0 0 1 2 2 2
  line L172 (27.3886, -19.3387) -> (27.7251, -18.8836)
  line L173 (27.7251, -18.8836) -> (24.2659, -16.3262)
  line L174 (24.2659, -16.3262) -> (23.9294, -16.7813)
  spline S167 degree 2 poles (23.9294, -16.7813) (23.6359, -17.1782) (23.3192, -17.8733) (23.31, -18.2438) knots 0 0 0 1 2 2 2
  spline S168 degree 2 poles (23.31, -18.2438) (23.2897, -18.7131) (23.7573, -19.5431) (24.2816, -19.9307) knots 0 0 0 1 2 2 2
  line L175 (22.3316, -22.5025) -> (22.959, -21.862)
  line L176 (22.959, -21.862) -> (23.7225, -22.6098)
  line L177 (23.7225, -22.6098) -> (23.095, -23.2504)
  line L178 (23.095, -23.2504) -> (22.3316, -22.5025)
  line L179 (20.0995, -20.3161) -> (20.7269, -19.6755)
  line L180 (20.7269, -19.6755) -> (21.4904, -20.4234)
  line L181 (21.4904, -20.4234) -> (20.8629, -21.0639)
  line L182 (20.8629, -21.0639) -> (20.0995, -20.3161)
  spline S169 degree 2 poles (18.8916, -27.8268) (19.0608, -27.7133) (19.3399, -27.406) (19.4587, -27.2335) knots 0 0 0 1 2 2 2
  spline S170 degree 2 poles (19.4587, -27.2335) (19.5663, -27.0687) (19.6973, -26.7844) (19.7434, -26.6662) knots 0 0 0 1 2 2 2
  line L183 (19.7434, -26.6662) -> (19.781, -26.641)
  line L184 (19.781, -26.641) -> (20.2226, -27.299)
  spline S171 degree 2 poles (20.2226, -27.299) (20.0927, -27.5443) (19.5156, -28.1879) (19.2035, -28.3973) knots 0 0 0 1 2 2 2
  spline S172 degree 2 poles (19.2035, -28.3973) (18.8877, -28.6093) (18.3319, -28.7968) (18.0493, -28.7902) knots 0 0 0 1 2 2 2
  spline S173 degree 2 poles (18.0493, -28.7902) (17.7478, -28.7798) (17.2521, -28.4962) (17.0603, -28.2104) knots 0 0 0 1 2 2 2
  spline S174 degree 2 poles (17.0603, -28.2104) (16.803, -27.8269) (16.9182, -26.9097) (17.2212, -26.5973) knots 0 0 0 1 2 2 2
  line L185 (17.2212, -26.5973) -> (17.1909, -26.5522)
  spline S175 degree 2 poles (17.1909, -26.5522) (17.0241, -26.6205) (16.5986, -26.7097) (16.3649, -26.6702) knots 0 0 0 1 2 2 2
  spline S176 degree 2 poles (16.3649, -26.6702) (16.1337, -26.6345) (15.6706, -26.3345) (15.4662, -26.0299) knots 0 0 0 1 2 2 2
  spline S177 degree 2 poles (15.4662, -26.0299) (15.2568, -25.7178) (15.1153, -25.0438) (15.1746, -24.7095) knots 0 0 0 1 2 2 2
  spline S178 degree 2 poles (15.1746, -24.7095) (15.2363, -24.3627) (15.6653, -23.7585) (16.03, -23.5138) knots 0 0 0 1 2 2 2
  spline S179 degree 2 poles (16.03, -23.5138) (16.3797, -23.2791) (17.1776, -22.9891) (17.489, -22.9492) knots 0 0 0 1 2 2 2
  line L186 (17.489, -22.9492) -> (17.9305, -23.6072)
  line L187 (17.9305, -23.6072) -> (17.8854, -23.6375)
  spline S180 degree 2 poles (17.8854, -23.6375) (17.594, -23.6258) (16.7556, -23.8067) (16.4284, -24.0263) knots 0 0 0 1 2 2 2
  spline S181 degree 2 poles (16.4284, -24.0263) (16.2367, -24.1549) (15.9339, -24.5326) (15.8994, -24.7576) knots 0 0 0 1 2 2 2
  spline S182 degree 2 poles (15.8994, -24.7576) (15.8687, -24.98) (15.9591, -25.3992) (16.1282, -25.6511) knots 0 0 0 1 2 2 2
  spline S183 degree 2 poles (16.1282, -25.6511) (16.2972, -25.903) (16.6634, -26.1318) (16.8581, -26.1375) knots 0 0 0 1 2 2 2
  spline S184 degree 2 poles (16.8581, -26.1375) (17.0528, -26.1431) (17.458, -25.9749) (17.6685, -25.8336) knots 0 0 0 1 2 2 2
  line L188 (17.6685, -25.8336) -> (17.9317, -25.6569)
  line L189 (17.9317, -25.6569) -> (18.2774, -26.1721)
  line L190 (18.2774, -26.1721) -> (18.0706, -26.3109)
  spline S185 degree 2 poles (18.0706, -26.3109) (17.6532, -26.5909) (17.3943, -27.3428) (17.6491, -27.7226) knots 0 0 0 1 2 2 2
  spline S186 degree 2 poles (17.6491, -27.7226) (17.7677, -27.8993) (18.0722, -28.0604) (18.2317, -28.0624) knots 0 0 0 1 2 2 2
  spline S187 degree 2 poles (18.2317, -28.0624) (18.4012, -28.0632) (18.7299, -27.9353) (18.8916, -27.8268) knots 0 0 0 1 2 2 2
  line L191 (12.7273, -25.5879) -> (13.5238, -25.1762)
  line L192 (13.5238, -25.1762) -> (14.0146, -26.1256)
  line L193 (14.0146, -26.1256) -> (13.2181, -26.5373)
  line L194 (13.2181, -26.5373) -> (12.7273, -25.5879)
  line L195 (8.5079, -27.3356) -> (11.7292, -26.1115)
  line L196 (11.7292, -26.1115) -> (12.0107, -26.8523)
  spline S188 degree 2 poles (12.0107, -26.8523) (11.7874, -27.3101) (11.3994, -28.1503) (11.227, -28.5888) knots 0 0 0 1 2 2 2
  spline S189 degree 2 poles (11.227, -28.5888) (10.8795, -29.4717) (10.7426, -30.4248) (10.9019, -30.8438) knots 0 0 0 1 2 2 2
  spline S190 degree 2 poles (10.9019, -30.8438) (10.9855, -31.064) (11.2465, -31.3427) (11.4094, -31.4018) knots 0 0 0 1 2 2 2
  spline S191 degree 2 poles (11.4094, -31.4018) (11.5724, -31.461) (11.9343, -31.4446) (12.129, -31.3706) knots 0 0 0 1 2 2 2
  spline S192 degree 2 poles (12.129, -31.3706) (12.3153, -31.2998) (12.6609, -31.0619) (12.8071, -30.924) knots 0 0 0 1 2 2 2
  spline S193 degree 2 poles (12.8071, -30.924) (12.9327, -30.8085) (13.1435, -30.5346) (13.2057, -30.4432) knots 0 0 0 1 2 2 2
  line L197 (13.2057, -30.4432) -> (13.2438, -30.4287)
  line L198 (13.2438, -30.4287) -> (13.5269, -31.1737)
  spline S194 degree 2 poles (13.5269, -31.1737) (13.3512, -31.3616) (12.6554, -31.8633) (12.3083, -31.9952) knots 0 0 0 1 2 2 2
  spline S195 degree 2 poles (12.3083, -31.9952) (11.576, -32.2735) (10.4561, -31.8125) (10.2052, -31.1522) knots 0 0 0 1 2 2 2
  spline S196 degree 2 poles (10.2052, -31.1522) (10.0878, -30.8432) (10.0355, -30.272) (10.0788, -30.0037) knots 0 0 0 1 2 2 2
  spline S197 degree 2 poles (10.0788, -30.0037) (10.1189, -29.7268) (10.3167, -29.1382) (10.4379, -28.8451) knots 0 0 0 1 2 2 2
  spline S198 degree 2 poles (10.4379, -28.8451) (10.6313, -28.3598) (11.1471, -27.2822) (11.3031, -26.9661) knots 0 0 0 1 2 2 2
  line L199 (11.3031, -26.9661) -> (8.7379, -27.9409)
  line L200 (8.7379, -27.9409) -> (8.5079, -27.3356)
  spline S199 degree 2 poles (4.8659, -30.0056) (4.7793, -29.612) (4.8834, -28.8843) (5.0589, -28.586) knots 0 0 0 1 2 2 2
  spline S200 degree 2 poles (5.0589, -28.586) (5.2343, -28.2877) (5.8565, -27.8494) (6.2811, -27.7559) knots 0 0 0 1 2 2 2
  spline S201 degree 2 poles (6.2811, -27.7559) (6.6703, -27.6703) (7.4689, -27.6753) (7.7777, -27.7511) knots 0 0 0 1 2 2 2
  line L201 (7.7777, -27.7511) -> (7.9481, -28.525)
  line L202 (7.9481, -28.525) -> (7.895, -28.5367)
  spline S202 degree 2 poles (7.895, -28.5367) (7.7973, -28.4933) (7.4483, -28.4032) (7.2425, -28.3743) knots 0 0 0 1 2 2 2
  spline S203 degree 2 poles (7.2425, -28.3743) (7.0093, -28.3468) (6.6326, -28.3416) (6.407, -28.3913) knots 0 0 0 1 2 2 2
  spline S204 degree 2 poles (6.407, -28.3913) (6.1859, -28.4399) (5.8052, -28.6907) (5.6928, -28.8962) knots 0 0 0 1 2 2 2
  spline S205 degree 2 poles (5.6928, -28.8962) (5.5918, -29.09) (5.5456, -29.5546) (5.6099, -29.8465) knots 0 0 0 1 2 2 2
  spline S206 degree 2 poles (5.6099, -29.8465) (5.6741, -30.1384) (5.9151, -30.4748) (6.0927, -30.5655) knots 0 0 0 1 2 2 2
  spline S207 degree 2 poles (6.0927, -30.5655) (6.2777, -30.6686) (6.7629, -30.6823) (7.0416, -30.621) knots 0 0 0 1 2 2 2
  spline S208 degree 2 poles (7.0416, -30.621) (7.3423, -30.5548) (7.9189, -30.3305) (8.0914, -30.2508) knots 0 0 0 1 2 2 2
  line L203 (8.0914, -30.2508) -> (8.7106, -33.0635)
  line L204 (8.7106, -33.0635) -> (5.7165, -33.7225)
  line L205 (5.7165, -33.7225) -> (5.5754, -33.0813)
  line L206 (5.5754, -33.0813) -> (7.8662, -32.577)
  line L207 (7.8662, -32.577) -> (7.546, -31.122)
  spline S209 degree 2 poles (7.546, -31.122) (7.4172, -31.1689) (7.1636, -31.2386) (7.0575, -31.262) knots 0 0 0 1 2 2 2
  spline S210 degree 2 poles (7.0575, -31.262) (6.6373, -31.3545) (6.0278, -31.3449) (5.7177, -31.1999) knots 0 0 0 1 2 2 2
  spline S211 degree 2 poles (5.7177, -31.1999) (5.4031, -31.0558) (4.975, -30.5009) (4.8659, -30.0056) knots 0 0 0 1 2 2 2
  line L208 (1.9644, -34.3741) -> (1.9325, -32.1946)
  line L209 (1.9325, -32.1946) -> (2.4241, -32.1505)
  line L210 (2.4241, -32.1505) -> (2.7807, -34.3008)
  line L211 (2.7807, -34.3008) -> (1.9644, -34.3741)
  line L212 (3.3716, -34.2478) -> (3.3397, -32.0683)
  line L213 (3.3397, -32.0683) -> (3.8313, -32.0242)
  line L214 (3.8313, -32.0242) -> (4.1879, -34.1745)
  line L215 (4.1879, -34.1745) -> (3.3716, -34.2478)
  line L216 (-5.9653, -28.0189) -> (-5.2298, -28.1218)
  line L217 (-5.2298, -28.1218) -> (-5.6085, -30.8306)
  line L218 (-5.6085, -30.8306) -> (-3.0612, -31.1867)
  line L219 (-3.0612, -31.1867) -> (-2.6825, -28.4779)
  line L220 (-2.6825, -28.4779) -> (-1.947, -28.5807)
  line L221 (-1.947, -28.5807) -> (-2.7206, -34.1149)
  line L222 (-2.7206, -34.1149) -> (-3.4561, -34.0121)
  line L223 (-3.4561, -34.0121) -> (-3.1527, -31.8414)
  line L224 (-3.1527, -31.8414) -> (-5.7, -31.4853)
  line L225 (-5.7, -31.4853) -> (-6.0035, -33.6559)
  line L226 (-6.0035, -33.6559) -> (-6.739, -33.5531)
  line L227 (-6.739, -33.5531) -> (-5.9653, -28.0189)
  spline S212 degree 2 poles (-8.1967, -27.2935) (-7.6431, -27.4494) (-7.1977, -28.2569) (-7.3904, -28.9412) knots 0 0 0 1 2 2 2
  line L228 (-7.3904, -28.9412) -> (-8.0199, -31.1774)
  line L229 (-8.0199, -31.1774) -> (-7.5623, -31.3062)
  line L230 (-7.5623, -31.3062) -> (-7.7206, -31.8685)
  line L231 (-7.7206, -31.8685) -> (-8.1783, -31.7397)
  line L232 (-8.1783, -31.7397) -> (-8.5047, -32.8991)
  line L233 (-8.5047, -32.8991) -> (-9.1847, -32.7077)
  line L234 (-9.1847, -32.7077) -> (-8.8582, -31.5482)
  line L235 (-8.8582, -31.5482) -> (-10.1093, -31.196)
  line L236 (-10.1093, -31.196) -> (-9.9509, -30.6337)
  line L237 (-9.9509, -30.6337) -> (-8.6999, -30.9859)
  line L238 (-8.6999, -30.9859) -> (-8.1588, -29.0637)
  spline S213 degree 2 poles (-8.1588, -29.0637) (-8.0729, -28.7585) (-8.0002, -28.4168) (-8.0338, -28.2521) knots 0 0 0 1 2 2 2
  spline S214 degree 2 poles (-8.0338, -28.2521) (-8.0592, -28.1085) (-8.2982, -27.9047) (-8.5336, -27.8385) knots 0 0 0 1 2 2 2
  spline S215 degree 2 poles (-8.5336, -27.8385) (-8.6992, -27.7918) (-9.037, -27.805) (-9.1153, -27.8158) knots 0 0 0 1 2 2 2
  line L239 (-9.1153, -27.8158) -> (-9.1545, -27.8048)
  line L240 (-9.1545, -27.8048) -> (-8.9827, -27.1946)
  spline S216 degree 2 poles (-8.9827, -27.1946) (-8.7762, -27.1962) (-8.3667, -27.2457) (-8.1967, -27.2935) knots 0 0 0 1 2 2 2
  line L241 (-11.7901, -29.4288) -> (-10.9532, -29.7505)
  line L242 (-10.9532, -29.7505) -> (-11.3365, -30.7481)
  line L243 (-11.3365, -30.7481) -> (-12.1735, -30.4264)
  line L244 (-12.1735, -30.4264) -> (-11.7901, -29.4288)
  line L245 (-10.6692, -26.5122) -> (-9.8323, -26.8339)
  line L246 (-9.8323, -26.8339) -> (-10.2157, -27.8315)
  line L247 (-10.2157, -27.8315) -> (-11.0526, -27.5098)
  line L248 (-11.0526, -27.5098) -> (-10.6692, -26.5122)
  line L249 (-16.9361, -23.0822) -> (-14.0378, -24.9464)
  line L250 (-14.0378, -24.9464) -> (-14.4665, -25.6129)
  spline S217 degree 2 poles (-14.4665, -25.6129) (-14.9675, -25.7053) (-15.8738, -25.8922) (-16.329, -26.014) knots 0 0 0 1 2 2 2
  spline S218 degree 2 poles (-16.329, -26.014) (-17.2458, -26.2589) (-18.0937, -26.715) (-18.3362, -27.092) knots 0 0 0 1 2 2 2
  spline S219 degree 2 poles (-18.3362, -27.092) (-18.4636, -27.2901) (-18.5328, -27.6655) (-18.4836, -27.8318) knots 0 0 0 1 2 2 2
  spline S220 degree 2 poles (-18.4836, -27.8318) (-18.4344, -27.998) (-18.2062, -28.2794) (-18.031, -28.3921) knots 0 0 0 1 2 2 2
  spline S221 degree 2 poles (-18.031, -28.3921) (-17.8634, -28.4999) (-17.4668, -28.6366) (-17.269, -28.6723) knots 0 0 0 1 2 2 2
  spline S222 degree 2 poles (-17.269, -28.6723) (-17.1014, -28.7047) (-16.7558, -28.7116) (-16.6454, -28.7073) knots 0 0 0 1 2 2 2
  line L251 (-16.6454, -28.7073) -> (-16.6111, -28.7293)
  line L252 (-16.6111, -28.7293) -> (-17.0422, -29.3996)
  spline S223 degree 2 poles (-17.0422, -29.3996) (-17.2977, -29.3699) (-18.1147, -29.1082) (-18.427, -28.9073) knots 0 0 0 1 2 2 2
  spline S224 degree 2 poles (-18.427, -28.9073) (-19.0859, -28.4835) (-19.3802, -27.3089) (-18.9981, -26.7147) knots 0 0 0 1 2 2 2
  spline S225 degree 2 poles (-18.9981, -26.7147) (-18.8193, -26.4367) (-18.3909, -26.0554) (-18.1493, -25.9308) knots 0 0 0 1 2 2 2
  spline S226 degree 2 poles (-18.1493, -25.9308) (-17.9027, -25.7987) (-17.3117, -25.6081) (-17.004, -25.5314) knots 0 0 0 1 2 2 2
  spline S227 degree 2 poles (-17.004, -25.5314) (-16.4987, -25.3988) (-15.3254, -25.1735) (-14.9785, -25.1113) knots 0 0 0 1 2 2 2
  line L253 (-14.9785, -25.1113) -> (-17.2864, -23.6268)
  line L254 (-17.2864, -23.6268) -> (-16.9361, -23.0822)
  line L255 (-18.4342, -21.8382) -> (-17.7401, -22.4059)
  line L256 (-17.7401, -22.4059) -> (-18.4167, -23.2331)
  line L257 (-18.4167, -23.2331) -> (-19.1108, -22.6655)
  line L258 (-19.1108, -22.6655) -> (-18.4342, -21.8382)
  line L259 (-25.1632, -21.9249) -> (-20.0716, -20.3474)
  line L260 (-20.0716, -20.3474) -> (-19.5161, -20.9188)
  line L261 (-19.5161, -20.9188) -> (-24.8322, -22.5252)
  line L262 (-24.8322, -22.5252) -> (-22.8215, -24.5934)
  line L263 (-22.8215, -24.5934) -> (-23.2923, -25.0511)
  line L264 (-23.2923, -25.0511) -> (-25.7639, -22.5088)
  line L265 (-25.7639, -22.5088) -> (-25.1632, -21.9249)
  spline S228 degree 2 poles (-25.6093, -16.3761) (-25.2824, -16.1403) (-24.5732, -15.947) (-24.2298, -15.9897) knots 0 0 0 1 2 2 2
  spline S229 degree 2 poles (-24.2298, -15.9897) (-23.8864, -16.0323) (-23.237, -16.4295) (-22.9828, -16.782) knots 0 0 0 1 2 2 2
  spline S230 degree 2 poles (-22.9828, -16.782) (-22.7496, -17.1053) (-22.4373, -17.8403) (-22.3843, -18.1538) knots 0 0 0 1 2 2 2
  line L266 (-22.3843, -18.1538) -> (-23.027, -18.6173)
  line L267 (-23.027, -18.6173) -> (-23.0588, -18.5733)
  spline S231 degree 2 poles (-23.0588, -18.5733) (-23.0577, -18.4664) (-23.1135, -18.1103) (-23.1687, -17.91) knots 0 0 0 1 2 2 2
  spline S232 degree 2 poles (-23.1687, -17.91) (-23.236, -17.685) (-23.3808, -17.3371) (-23.5159, -17.1498) knots 0 0 0 1 2 2 2
  spline S233 degree 2 poles (-23.5159, -17.1498) (-23.6484, -16.9662) (-24.0296, -16.7163) (-24.2629, -16.6947) knots 0 0 0 1 2 2 2
  spline S234 degree 2 poles (-24.2629, -16.6947) (-24.4809, -16.6789) (-24.9256, -16.8209) (-25.168, -16.9958) knots 0 0 0 1 2 2 2
  spline S235 degree 2 poles (-25.168, -16.9958) (-25.4104, -17.1706) (-25.6235, -17.5253) (-25.6363, -17.7244) knots 0 0 0 1 2 2 2
  spline S236 degree 2 poles (-25.6363, -17.7244) (-25.6575, -17.935) (-25.4775, -18.3859) (-25.3106, -18.6173) knots 0 0 0 1 2 2 2
  spline S237 degree 2 poles (-25.3106, -18.6173) (-25.1305, -18.867) (-24.6957, -19.3072) (-24.5541, -19.4339) knots 0 0 0 1 2 2 2
  line L268 (-24.5541, -19.4339) -> (-26.89, -21.1186)
  line L269 (-26.89, -21.1186) -> (-28.6833, -18.6321)
  line L270 (-28.6833, -18.6321) -> (-28.1507, -18.2481)
  line L271 (-28.1507, -18.2481) -> (-26.7786, -20.1506)
  line L272 (-26.7786, -20.1506) -> (-25.5703, -19.2791)
  spline S238 degree 2 poles (-25.5703, -19.2791) (-25.6644, -19.1795) (-25.8291, -18.9744) (-25.8926, -18.8863) knots 0 0 0 1 2 2 2
  spline S239 degree 2 poles (-25.8926, -18.8863) (-26.1443, -18.5374) (-26.3774, -17.9741) (-26.3674, -17.6319) knots 0 0 0 1 2 2 2
  spline S240 degree 2 poles (-26.3674, -17.6319) (-26.36, -17.286) (-26.0207, -16.6728) (-25.6093, -16.3761) knots 0 0 0 1 2 2 2
  line L273 (-30.7706, -15.4468) -> (-28.7828, -14.5524)
  line L274 (-28.7828, -14.5524) -> (-28.5472, -14.9862)
  line L275 (-28.5472, -14.9862) -> (-30.3793, -16.1671)
  line L276 (-30.3793, -16.1671) -> (-30.7706, -15.4468)
  line L277 (-30.0961, -16.6883) -> (-28.1084, -15.7939)
  line L278 (-28.1084, -15.7939) -> (-27.8727, -16.2276)
  line L279 (-27.8727, -16.2276) -> (-29.7049, -17.4085)
  line L280 (-29.7049, -17.4085) -> (-30.0961, -16.6883)
  dimension "d145" = 57.15
  constraints: 1 centre point, 1 coincident, 1 other
  measures "d145" diameter of A0
extrude "Extrusion19" cut sketch "Sketch26" against normal blind 1.27
equation "\"d85\" = spoolExteriorRadius"
equation "\"d86\" = spoolOverallHeight"
equation "\"d88\" = d85"
equation "\"d89\" = 0.5 * spoolOverallHeight"
equation "\"centerLineForSpool\" = 0.25 * spoolOverallHeight"
equation "\"d103\" = hexDiameter"
equation "\"d110\" = centerLineForSpool"
equation "\"d111\" = centerLineForSpool"
equation "\"d112\" = holeForString"
equation "\"d121\" = centerLineForSpool"
equation "\"d122\" = holeForString"
equation "\"d125\" = knotHoleDiameter"
equation "\"d127\" = holeForString"
equation "\"d128\" = centerLineForSpool"
equation "\"d129\" = knotHoleDiameter"
equation "\"d130\" = knotHoleDepth"
equation "\"d132\" = hexHoleChamfer"
equation "\"holeForString\" = stringDiameter + clearanceForString"
equation "\"stringDiameter\" = 3.048"
equation "\"clearanceForString\" = 2.032"
equation "\"spoolHeightWithoutSpacer\" = 69.85"
equation "\"hexShaftDiameter\" = 12.7"
equation "\"clearanceForHexShaft\" = 0.5715"
equation "\"hexDiameter\" = hexShaftDiameter + clearanceForHexShaft"
equation "\"supportChannels\" = 3.81"
equation "\"spoolInteriorDiameter\" = 38.1"
equation "\"spoolInteriroRadius\" = 0.5 * spoolInteriorDiameter"
equation "\"spoolExteriorDiameter\" = 82.55"
equation "\"spoolExteriorRadius\" = 0.5 * spoolExteriorDiameter"
equation "\"spoolFiletRadius\" = 0.5 * supportChannels"
equation "\"holeCenter\" = 0.25 * spoolHeightWithoutSpacer - 0.75 * supportChannels"
equation "\"hexHoleChamfer\" = 1.5875"
equation "\"textCircleDiameter\" = 0.75 * spoolExteriorDiameter"
equation "\"textHeight\" = 6.096"
equation "\"textDepth\" = 1.27"
equation "\"stringHoleChamfer\" = 4.7625"
equation "\"spoolTotalHeight\" = 76.2"
equation "\"spaceHeight\" = spoolTotalHeight - spoolHeightWithoutSpacer"
equation "\"spacerDiameter\" = 24.13"
equation "\"spoolOverallHeight\" = 69.85"
equation "\"d114\" = -spoolInteriroRadius"
equation "\"knotHoleDiameter\" = 9.525"
equation "\"d126\" = spoolInteriroRadius"
equation "\"d141\" = -0.5 * spoolTotalHeight"
equation "\"knotHoleDepth\" = 11.1125"
body "Solid3"
